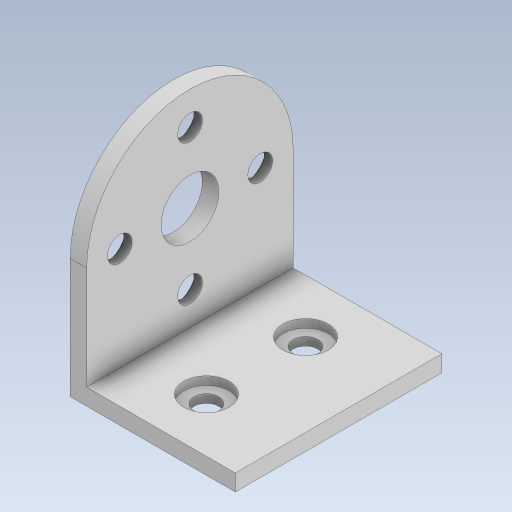
# Autodesk Inventor part: Bracket Motor JGA Depan
Saved by Autodesk Inventor 2023.5 (Build 275446000, 446)
## iProperties
Created: 2025-09-12
Part Number: Bracket Motor JGA Depan
Material: Generic
Document SubType Name: Modeling
Designer: Guntur
Density: 1 g/cm^3
Appearance: Default
Author: Guntur
Autodesk Inventor part; units mm, degrees
ref_plane "YZ Plane" through (0, 0, 0) normal (1, 0, 0) x (0, 1, 0)
ref_plane "XZ Plane" through (0, 0, 0) normal (0, 1, 0) x (-1, 0, 0)
ref_plane "XY Plane" through (0, 0, 0) normal (0, 0, 1) x (1, 0, 0)
sketch "Sketch1" plane through (0, 0, 0) normal (0, 1, 0) x (-1, 0, 0)
  line L0 (10, 12.5) -> (-10, 12.5)
  line L1 (-10, 12.5) -> (-10, -12.5)
  line L2 (-10, -12.5) -> (10, -12.5)
  line L3 (10, -12.5) -> (10, 12.5)
  line L4 (10, 0) -> (-10, 0) construction
  line L5 (0, 12.5) -> (0, -12.5) construction
  line L6 (10, 12.5) -> (8, 12.5)
  line L7 (8, 12.5) -> (8, -12.5)
  line L8 (8, -12.5) -> (10, -12.5)
  line L9 (10, -12.5) -> (10, 12.5)
  circle A0 centre (0, 6) radius 1.5
  circle A1 centre (0, 6) radius 2.75
  circle A2 centre (0, -6) radius 1.5
  circle A3 centre (0, -6) radius 2.75
  point P0 (0, 0)
  point P1 (0, 0)
  dimension "d0" = 20
  dimension "d1" = 25
  dimension "d2" = 2
  dimension "d3" = 3
  dimension "d4" = 5.5
  dimension "d5" = 6
  constraints: 20 end point, 5 midpoint, 4 centre point, 4 parallel, 2 coincident, 2 horizontal, 2 perpendicular, 2 point on line, 2 symmetric about line, 2 other
  measures "d0" distance of L2.end L1.end
  measures "d1" distance of L1.end L0.end
  measures "d2" distance of L8.end L7.end
  measures "d3" diameter of A0
  measures "d4" diameter of A1
  measures "d5" distance of point (0, 0) A0.centre
extrude "Extrusion1" add sketch "Sketch1" along normal blind 2 contours L7 L2 L1 L0
extrude "Extrusion2" add sketch "Sketch1" along normal blind 1 contours A1 | A3
extrude "Extrusion3" add sketch "Sketch1" along normal blind 27 contours L3 L2 L7 L0
sketch "Sketch2" plane through (-8, 2, -12.5) normal (1, 0, 0) x (0, 0, -1)
  circle A0 centre (-12.5, 12.5) radius 12.5
  line L0 (-25, 25) -> (0, 25) projected
  line L1 (-12.5, 25) -> (-25, 25)
  line L2 (-25, 25) -> (-25, 12.5)
  line L3 (-25, 0) -> (-25, 25) projected
  line L4 (-12.5, 25) -> (0, 25)
  line L5 (0, 25) -> (0, 12.5)
  line L6 (0, 0) -> (0, 25) projected
  point P0 (-12.5, -2)
  point P1 (-25, 12.5)
  dimension "d12" = 25
  constraints: 8 end point, 3 midpoint, 1 centre point, 1 horizontal, 1 point on line, 1 tangent
  measures "d12" diameter of A0
extrude "Extrusion4" cut sketch "Sketch2" against normal blind 2 contours A0 L0 L5 | A0 L2 L0
sketch "Sketch3" plane through (-10, 0, -12.5) normal (-1, 0, 0) x (0, 0, 1)
  arc A0 (25, 14.5) -> (0, 14.5) centre (12.5, 14.5) ccw projected
  circle A1 centre (21, 14.5) radius 1.5
  circle A2 centre (21, 14.5) radius 2.75
  line L0 (12.5, 14.5) -> (12.5, 17.4625)
  circle A3 centre (4, 14.5) radius 1.5
  circle A4 centre (4, 14.5) radius 2.75
  circle A5 centre (12.5, 14.5) radius 3.5
  circle A6 centre (12.5, 6) radius 1.5
  circle A7 centre (12.5, 6) radius 2.75
  circle A8 centre (12.5, 23) radius 1.5
  circle A9 centre (12.5, 23) radius 2.75
  point P0 (12.5, 0)
  dimension "d15" = 3
  dimension "d16" = 5.5
  dimension "d17" = 8.5
  dimension "d22" = 7
  dimension "d25" = 3
  dimension "d26" = 5.5
  dimension "d27" = 8.5
  dimension "d28" = 3
  dimension "d29" = 5.5
  dimension "d30" = 8.5
  constraints: 9 centre point, 5 coincident, 2 end point, 2 symmetric about line, 1 vertical, 2 other
  measures "d15" diameter of A1
  measures "d16" diameter of A2
  measures "d17" distance from line of L0 A1.centre
  measures "d22" diameter of A5
  measures "d25" diameter of A6
  measures "d26" diameter of A7
  measures "d27" distance of A6.centre L0.start
  measures "d28" diameter of A8
  measures "d29" diameter of A9
  measures "d30" distance of L0.start A9.centre
extrude "Extrusion5" cut sketch "Sketch3" against normal blind 2 contours A1 | A3 | A6 | A8
extrude "Extrusion6" cut sketch "Sketch3" against normal blind 1 contours A2 | A4 | A7 | A9
extrude "Extrusion7" cut sketch "Sketch3" against normal blind 2 contours A5
body "Solid1"
